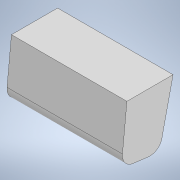
# Autodesk Inventor part: hook thing
Saved by Autodesk Inventor 2020.2 (Build 242310000, 310)
## iProperties
Created: 2020-05-05
Part Number: hook thing
Material: Generic
Document SubType Name: Modeling
Designer: Amaan Khalid
Density: 1 g/cm^3
Appearance: Default
Author: Amaan Khalid
Autodesk Inventor part; units mm, degrees
ref_plane "YZ Plane" through (0, 0, 0) normal (1, 0, 0) x (0, 1, 0)
ref_plane "XZ Plane" through (0, 0, 0) normal (0, 1, 0) x (-1, 0, 0)
ref_plane "XY Plane" through (0, 0, 0) normal (0, 0, 1) x (1, 0, 0)
sketch "Sketch1" plane through (0, 0, 0) normal (1, 0, 0) x (0, 1, 0)
  line L0 (-25.4, -0.407) -> (-25.4, 4.334)
  line L1 (-31.4459, 2.1226) -> (-31.2483, 3.6877)
  line L2 (-29.8585, 4.792) -> (-25.4, 4.334)
  arc A0 (-29.8585, 4.792) -> (-31.2483, 3.6877) centre (-29.9883, 3.5287) ccw
  arc A1 (-31.4459, 2.1226) -> (-30.2966, 0.6984) centre (-30.1859, 1.9636) ccw
  line L3 (-25.4, 0) -> (-25.4, 4.064)
  line L4 (-25.4, -0.407) -> (-30.2966, 0.6984)
  point P0 (0, 0)
  dimension "d1" = 1.27
  dimension "d6" = 4.741
  constraints: 10 end point, 4 point on circle, 3 tangent, 2 centre point, 1 equal radius
  measures "d1" radius of A0
  measures "d6" distance of L0.start L0.end
extrude "Extrusion1" add sketch "Sketch1" along normal blind 11.8618
body "Solid1"
